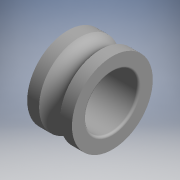
# Autodesk Inventor part: 607ZZ Inner ring
Saved by Autodesk Inventor 2017.3 (Build 213256000, 256)
## iProperties
Part Number: 607ZZ Inner ring
Material: Generic
Catalog Web Link: www.cadenas.de
Description: Six types ir-Metric system sizes
Vendor: NTN
Document SubType Name: Modeling
Designer: partserver
Manufacturer: NTN
Mass: 0.277743 g
Surface Area: 4.43852 cm^2
Volume: 0.277743 cm^3
Density: 1 g/cm^3
Appearance: PSOLRGB-192-192-192
Category: PARTsolutions
Company: NTN
Title: 607ZZ Inner ring
Author: Cadenas PARTsolutions
Comments: Metric system sizes
PSOL_IDENT_0: {$CADENAS_DATA\23d-libs\ntn\ball_roller_bearings\miniature_extra_small_bb\metric_system_sizes\mss_ir
PSOL_IDENT_1: .prj},181 {VTYP=3D},{NB=607ZZ Inner ring},{LINA=607ZZ Inner ring},{NN=Six types ir},{DATE=21.12.2021
PSOL_IDENT_2: 04:23:04},{GEOMDATE=06.03.2020 10:06:06},{VERSION=},{LINEID=12950},{WBVAR=},{WBNUMERIC=}  {NB=607ZZ
PSOL_IDENT_3: Inner ring},{LINA=607ZZ Inner ring},{KT=DUMMY},{IDNR=},{SD=7.0},{D=19},{B=6.0},{R=0.30},{ORDER=607Z
PSOL_IDENT_4: Z},{CR=2 240},{COR=910},{CRF=228},{CORF=93},{LSG=34 000},{LSO=40 000},{MASS=8.00},{D1=0.0},{D2=0.0},
PSOL_IDENT_5: {C1=0.0},{C2=0.0},{ORDER1=607},{WSS=607ZZ},{WDS=ZZ},{UTWF=0},{FORSS=0},{FORDS=0},{DA1=9},{DA2=10,4},
PSOL_IDENT_6: {DA=17},{RAS=0,3},{MASS1=0.00},{B1=6.0},{VERS=3},{X=6},{N=7},{O=40.82},{RB=1.776}
NB: 607ZZ Inner ring
NN: Six types ir
NT: Metric system sizes
NBSYN: $ORDER. Inner ring
LINA: 607ZZ Inner ring
CATALOG: NTN Corporation
SD: 7
D: 19
B: 6
R: 0.3
CR: 2 240
COR: 910
CRF: 228
CORF: 93
LSG: 34 000
LSO: 40 000
MASS: 8
D1: 0
D2: 0
C1: 0
C2: 0
ORDER1: 607
WSS: 607ZZ
WDS: ZZ
UTWF: 0
FORSS: 0
FORDS: 0
DA1: 9
DA2: 10,4
DA: 17
RAS: 0,3
MASS1: 0
B1: 6
VERS: 3
SUPPLIER: NTN
ARTICLENO: 607ZZ Inner ring
BOMINFO: 607ZZ Inner ring
CREATOR: CADENAS GmbH
Autodesk Inventor part; units mm, degrees
sketch "Sketch_2" plane through (0, 0, 0) normal (0, 0, 1) x (1, 0, 0)
  line L0 (6, 0) -> (0, 0)
  arc A0 (0, 3.8) -> (0.3, 3.5) centre (0.3, 3.8) ccw
  line L1 (0.3, 3.5) -> (5.7, 3.5)
  arc A1 (5.7, 3.5) -> (6, 3.8) centre (5.7, 3.8) ccw
  line L2 (6, 3.8) -> (6, 5.42)
  line L3 (6, 5.42) -> (4.4099, 5.42)
  arc A2 (1.5901, 5.42) -> (4.4099, 5.42) centre (3, 6.5) ccw
  line L4 (1.5901, 5.42) -> (0, 5.42)
  line L5 (0, 5.42) -> (0, 3.8)
  constraints: 12 end point, 6 point on circle, 3 centre point
revolve "Revolution1" add sketch "Sketch_2" angle 360 about axis through (6, 0, 0) along (1, 0, 0)
ref_plane "mss_ir_XY" through (0, 0, 0) normal (1, 0, 0) x (0, 0, -1)
ref_plane "mss_ir_YZ" through (0, 0, 0) normal (0, 0, -1) x (0, 1, 0)
ref_plane "mss_ir_ZX" through (0, 0, 0) normal (0, 1, 0) x (1, 0, 0)
body "Solid1"
